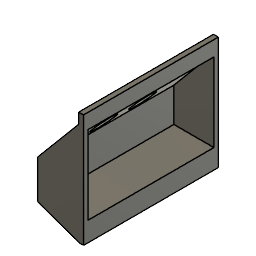
Plataforma para Sensor (Autodesk Fusion 360 design; units mm, degrees)
part number: 2026-06-29-13-53-25-750
Autodesk Fusion 360 part; units mm, degrees
sketch "Boceto1" plane through (0, 0, 0) normal (0, 1, 0) x (1, 0, 0)
  line L0 (0, 0) -> (45.0979, 0)
  line L1 (45.0979, 0) -> (45.0979, -89.5)
  line L2 (45.0979, -89.5) -> (0, -89.5)
  line L3 (0, -89.5) -> (0, 0)
  dimension "d1" = 89.5
  constraint horizontal L0
  constraint vertical L1
  constraint horizontal L2
  constraint vertical L3
  constraint coincident L0.start L3.end
  measures "d1" distance of L0.start L2.end
extrude "Extruir1" add sketch "Boceto1" along normal blind 3
sketch "Boceto2" plane through (0, 0, 0) normal (0, -1, 0) x (1, 0, 0)
  line L0 (45.0979, 89.5) -> (0, 89.5)
  line L1 (0, 89.5) -> (0, 0)
  line L2 (0, 0) -> (45.0979, 0)
  line L3 (45.0979, 0) -> (45.0979, 89.5)
  line L4 (0, 0) -> (12.1, 0)
  line L5 (12.1, 89.5) -> (0, 89.5)
  line L6 (0, 89.5) -> (0, 0)
  point P0 (12.1, 0)
  point P1 (12.1, 89.5)
  constraint horizontal L4
  constraint horizontal L5
  constraint vertical L6
  constraint coincident L1.end L2.start
  constraint coincident P0 L4.end
  constraint coincident P1 L5.start
ref_plane "PlanoDeObra1" through (12.1, 0, 44.75) normal (-0.707107, 0.707107, 0) x (0, 0, -1)
sketch "Boceto3" plane through (45.0979, 0, 0) normal (1, 0, 0) x (0, 0, -1)
  line L0 (-89.5, 0) -> (0, 0)
  line L1 (0, 0) -> (0, 3)
  line L2 (0, 3) -> (-89.5, 3)
  line L3 (-89.5, 3) -> (-89.5, 0)
  line L4 (0, 0) -> (-89.5, 0)
  line L5 (-89.5, 0) -> (-89.5, 35.5)
  line L6 (-89.5, 35.5) -> (0, 35.5)
  line L7 (0, 35.5) -> (0, 0)
  line L8 (-86.5, 3) -> (-86.5, 32.5)
  line L9 (-86.5, 32.5) -> (-3, 32.5)
  line L10 (-3, 32.5) -> (-3, 3)
  line L11 (-3, 3) -> (-86.5, 3)
  dimension "d6" = 89.5
  dimension "d7" = 35.5
  dimension "d8" = 3
  constraint horizontal L4
  constraint vertical L5
  constraint horizontal L6
  constraint vertical L7
  constraint coincident L0.end L1.start
  measures "d6" distance of L0.end L0.start
  measures "d7" distance of L0.end L6.end
extrude "Extruir2" add sketch "Boceto3" against normal blind 3 contours L2 L5 L6 L7 L8 L9 L10
sketch "Boceto4" plane through (6.05, -6.05, 0) normal (-0.707107, 0.707107, 0) x (0, 0, -1)
ref_plane "PlanoDeObra2" through (12.1, 0, 44.75) normal (-0.766044, 0.642788, 0) x (0, 0, -1)
sketch "Boceto5" plane through (7.1006, -5.9581, 0) normal (-0.766044, 0.642788, 0) x (0, 0, -1)
  line L0 (-89.5, -7.7775) -> (0, -7.7775)
  line L1 (0, -7.7775) -> (0, -54.0244)
  line L2 (0, -54.0244) -> (-89.5, -54.0244)
  line L3 (-89.5, -54.0244) -> (-89.5, -7.7775)
  dimension "d12" = 89.5
  constraint horizontal L0
  constraint vertical L1
  constraint horizontal L2
  constraint vertical L3
  measures "d12" distance of L0.start L0.end
extrude "Extruir3" add sketch "Boceto5" against normal blind 3
extrude "Extruir4" cut sketch "Boceto2" along normal blind 3
sketch "Boceto6" plane through (7.1006, -5.9581, 0) normal (-0.766044, 0.642788, 0) x (0, 0, 1)
  line L0 (0, 11.694) -> (89.5, 11.694)
  line L1 (89.5, 11.694) -> (89.5, 54.0244)
  line L2 (89.5, 54.0244) -> (0, 54.0244)
  line L3 (0, 54.0244) -> (0, 11.694)
  circle A0 centre (57.7, 26.8462) radius 7.95
  circle A1 centre (31.8, 26.8462) radius 7.95
  dimension "d18" = 15.9
  dimension "d19" = 25.9
  dimension "d20" = 15.9
  measures "d18" diameter of A0
  measures "d19" distance of A0.centre A1.centre
  measures "d20" diameter of A1
extrude "Extruir5" cut sketch "Boceto6" against normal blind 3 contours A0 | A1
sketch "Boceto7" plane through (0, 3, 0) normal (0, 1, 0) x (-1, 0, 0)
  line L0 (-14.6173, 89.5) -> (-14.6173, 0)
  line L1 (-14.6173, 0) -> (0, 0)
  line L2 (0, 0) -> (0, 89.5)
  line L3 (0, 89.5) -> (-14.6173, 89.5)
  circle A0 centre (-8, 5) radius 3.25
  circle A1 centre (-7.3086, 84.9016) radius 3.25
  dimension "d23" = 6.5
  dimension "d24" = 6.5
  measures "d23" diameter of A0
  measures "d24" diameter of A1
extrude "Extruir6" cut sketch "Boceto7" against normal blind 3 contours A0 | A1
sketch "Boceto8" plane through (0, 0, 89.5) normal (0, 0, 1) x (1, 0, 0)
  line L0 (18.5335, 3) -> (42.0979, 31.083)
  line L1 (42.0979, 31.083) -> (42.0979, 3)
  line L2 (42.0979, 3) -> (18.5335, 3)
  line L3 (12.1, 0) -> (16.0162, 0)
  line L4 (16.0162, 0) -> (45.0979, 0)
  line L5 (45.0979, 0) -> (45.0979, 35.5)
  line L6 (45.0979, 35.5) -> (42.0979, 35.5)
  line L7 (42.0979, 35.5) -> (42.0979, 35.1995)
  line L8 (42.0979, 35.1995) -> (41.8268, 35.427)
  line L9 (41.8268, 35.427) -> (14.6173, 3)
  line L10 (14.6173, 3) -> (0, 3)
  line L11 (0, 3) -> (0, 0)
  line L12 (0, 0) -> (12.1, 0)
  line L13 (18.5335, 3) -> (42.0979, 3)
  line L14 (42.0979, 31.083) -> (18.5335, 3)
  constraint coincident L0.start L2.end
  constraint coincident L1.end L2.start
  constraint coincident L0.end L1.start
extrude "Extruir7" add sketch "Boceto8" against normal blind 3 contours L0 L1 L2 L13 L14
sketch "Boceto9" plane through (0, 0, 0) normal (0, 0, -1) x (-1, 0, 0)
  line L0 (-16.0162, 0) -> (-12.1, 0)
  line L1 (-12.1, 0) -> (0, 0)
  line L2 (0, 0) -> (0, 3)
  line L3 (0, 3) -> (-14.6173, 3)
  line L4 (-14.6173, 3) -> (-41.8268, 35.427)
  line L5 (-41.8268, 35.427) -> (-42.0979, 35.1995)
  line L6 (-42.0979, 35.1995) -> (-42.0979, 35.5)
  line L7 (-42.0979, 35.5) -> (-45.0979, 35.5)
  line L8 (-45.0979, 35.5) -> (-45.0979, 0)
  line L9 (-45.0979, 0) -> (-16.0162, 0)
  line L10 (-18.5335, 3) -> (-42.0979, 3)
  line L11 (-42.0979, 3) -> (-42.0979, 31.083)
  line L12 (-42.0979, 31.083) -> (-18.5335, 3)
  line L13 (-42.0979, 3) -> (-18.5335, 3)
  line L14 (-42.0979, 31.083) -> (-42.0979, 3)
  constraint coincident L10.end L11.start
  constraint coincident L10.start L12.end
  constraint coincident L11.end L12.start
extrude "Extruir8" add sketch "Boceto9" against normal blind 3 contours L10 L11 L12 L13 L14
sketch "Boceto10" plane through (45.0979, 0, 0) normal (1, 0, 0) x (0, 0, -1)
  line L0 (-3, 3) -> (-86.5, 3)
  line L1 (-86.5, 3) -> (-86.5, 32.5)
  line L2 (-86.5, 32.5) -> (-3, 32.5)
  line L3 (-3, 32.5) -> (-3, 3)
  line L4 (0, 0) -> (0, 35.5)
  line L5 (0, 35.5) -> (-89.5, 35.5)
  line L6 (-89.5, 35.5) -> (-89.5, 0)
  line L7 (-89.5, 0) -> (0, 0)
  line L8 (0, 34) -> (-89.5, 34)
  line L9 (-89.5, 34) -> (-89.5, 49.617)
  line L10 (-89.5, 49.617) -> (0, 49.617)
  line L11 (0, 49.617) -> (0, 34)
  dimension "d31" = 89.5
  dimension "d32" = 15.617
  constraint horizontal L8
  constraint vertical L9
  constraint horizontal L10
  constraint vertical L11
  constraint coincident L4 L8.start
  measures "d31" distance of L8.start L8.end
  measures "d32" distance of L8.start L10.end
extrude "Extruir9" add sketch "Boceto10" against normal blind 3.271 contours L4 L5 L6 L8 L9 L11 | L5 L9 L10 L11
sketch "Boceto11" plane through (41.8269, 0, 0) normal (-1, 0, 0) x (0, 0, 1)
  line L0 (0, 35.4269) -> (89.5, 35.4269)
  line L1 (89.5, 35.4269) -> (89.5, 49.617)
  line L2 (89.5, 49.617) -> (0, 49.617)
  line L3 (0, 49.617) -> (0, 35.4269)
  circle A0 centre (82, 43) radius 3.25
  circle A1 centre (10, 43) radius 3.25
  dimension "d35" = 6.5
  dimension "d36" = 6.5
  measures "d35" diameter of A0
  measures "d36" diameter of A1
extrude "Extruir10" cut sketch "Boceto11" against normal blind 3.271 contours A0 | A1
extrude "Extruir11" cut 1 faces at (41.8269, 42.6813, 2.25) along direction (1, 0, 0) blind 3
extrude "Extruir12" cut 1 faces at (44.8269, 42.6813, 2.25) along direction (1, 0, 0) blind 1
sketch "Boceto12" plane through (45.0979, 0, 0) normal (1, 0, 0) x (0, 0, -1)
  line L0 (-3, 3) -> (-86.5, 3)
  line L1 (-86.5, 3) -> (-86.5, 32.5)
  line L2 (-86.5, 32.5) -> (-3, 32.5)
  line L3 (-3, 32.5) -> (-3, 3)
  line L4 (0, 35.4269) -> (-89.5, 35.4269)
  line L5 (-89.5, 35.4269) -> (-89.5, 0)
  line L6 (-89.5, 0) -> (0, 0)
  line L7 (0, 0) -> (0, 35.4269)
  line L8 (0, 35.4269) -> (0, 42.4269)
  line L9 (0, 42.4269) -> (-10, 42.4269)
  line L10 (-10, 42.4269) -> (-10, -32.5731)
  line L11 (-10, -32.5731) -> (0, -32.5731)
  line L12 (0, -32.5731) -> (0, 42.4269)
  dimension "d43" = 7
  dimension "d44" = 10
  dimension "d45" = 75
  constraint coincident L4.start L7.end
  constraint perpendicular L4 L8
  constraint horizontal L9
  constraint vertical L10
  constraint horizontal L11
  constraint vertical L12
  measures "d43" distance of L4.start L8.end
  measures "d44" distance of L8.end L9.end
  measures "d45" distance of L8.end L11.end
extrude "Extruir13" add sketch "Boceto12" against normal blind 3.271 contours L0 L2 L3 L4 L6 L7 L10 L12 | L0 L2 L3 L10 | L6 L10 L11 L12 | L4 L8 L9 L10 L12
sketch "Boceto13" plane through (45.0979, 0, 0) normal (1, 0, 0) x (0, 0, -1)
  line L0 (-10, 3) -> (-86.5, 3)
  line L1 (-86.5, 3) -> (-86.5, 32.5)
  line L2 (-86.5, 32.5) -> (-10, 32.5)
  line L3 (-10, 32.5) -> (-10, 3)
  line L4 (0, -32.5731) -> (0, 42.4269)
  line L5 (0, 42.4269) -> (-10, 42.4269)
  line L6 (-10, 42.4269) -> (-10, 35.4269)
  line L7 (-10, 35.4269) -> (-89.5, 35.4269)
  line L8 (-89.5, 35.4269) -> (-89.5, 0)
  line L9 (-89.5, 0) -> (-10, 0)
  line L10 (-10, 0) -> (-10, -32.5731)
  line L11 (-10, -32.5731) -> (0, -32.5731)
  line L12 (-89.5, 35.4269) -> (-89.5, 42.4269)
  line L13 (-89.5, 42.4269) -> (-79.5, 42.4269)
  line L14 (-79.5, 42.4269) -> (-79.5, -32.5731)
  line L15 (-79.5, -32.5731) -> (-89.5, -32.5731)
  line L16 (-89.5, -32.5731) -> (-89.5, 42.4269)
  dimension "d48" = 7
  dimension "d49" = 10
  dimension "d50" = 75
  constraint coincident L7.end L8.start
  constraint perpendicular L7 L12
  constraint horizontal L13
  constraint vertical L14
  constraint horizontal L15
  constraint vertical L16
  measures "d48" distance of L7.end L12.end
  measures "d49" distance of L12.end L13.end
  measures "d50" distance of L12.end L15.end
extrude "Extruir14" add sketch "Boceto13" against normal blind 3.271 contours L0 L1 L2 L7 L8 L9 L14 L16 | L0 L1 L2 L14 | L9 L14 L15 L16 | L7 L12 L13 L14 L16
sketch "Boceto14" plane through (45.0979, 0, 0) normal (1, 0, 0) x (0, 0, -1)
  line L0 (-79.5, 0) -> (-10, 0)
  line L1 (-10, 0) -> (-10, -32.5731)
  line L2 (-10, -32.5731) -> (0, -32.5731)
  line L3 (0, -32.5731) -> (0, 42.4269)
  line L4 (0, 42.4269) -> (-10, 42.4269)
  line L5 (-10, 42.4269) -> (-10, 35.4269)
  line L6 (-10, 35.4269) -> (-79.5, 35.4269)
  line L7 (-79.5, 35.4269) -> (-79.5, 42.4269)
  line L8 (-79.5, 42.4269) -> (-89.5, 42.4269)
  line L9 (-89.5, 42.4269) -> (-89.5, -32.5731)
  line L10 (-89.5, -32.5731) -> (-79.5, -32.5731)
  line L11 (-79.5, -32.5731) -> (-79.5, 0)
  line L12 (-79.5, 3) -> (-79.5, 32.5)
  line L13 (-79.5, 32.5) -> (-10, 32.5)
  line L14 (-10, 32.5) -> (-10, 3)
  line L15 (-10, 3) -> (-79.5, 3)
  line L16 (0, -32.5731) -> (-89.5, -32.5731)
  line L17 (-89.5, -32.5731) -> (-89.5, -22.5731)
  line L18 (-89.5, -22.5731) -> (0, -22.5731)
  line L19 (0, -22.5731) -> (0, -32.5731)
  line L20 (-89.5, 42.4269) -> (0, 42.4269)
  line L21 (0, 42.4269) -> (0, 35.4269)
  line L22 (0, 35.4269) -> (-89.5, 35.4269)
  line L23 (-89.5, 35.4269) -> (-89.5, 42.4269)
  dimension "d53" = 10
  constraint horizontal L16
  constraint vertical L17
  constraint horizontal L18
  constraint vertical L19
  constraint coincident L2.end L3.start
  constraint horizontal L20
  constraint vertical L21
  constraint horizontal L22
  constraint vertical L23
  constraint coincident L3 L21.end
  constraint coincident L8.end L9.start
  measures "d53" distance of L2.end L18.end
extrude "Extruir15" add sketch "Boceto14" against normal blind 3.271 contours L1 L11 L16 L18 | L5 L6 L7 L20 L22
sketch "Boceto15" plane through (0, 3, 0) normal (0, 1, 0) x (-1, 0, 0)
  circle A0 centre (-7.3086, 84.9016) radius 3.25
  circle A1 centre (-8, 5) radius 3.25
  line L0 (-14.6173, 89.5) -> (-14.6173, 0)
  line L1 (-14.6173, 0) -> (0, 0)
  line L2 (0, 0) -> (0, 89.5)
  line L3 (0, 89.5) -> (-14.6173, 89.5)
  line L4 (0, 0) -> (-14.6173, 0)
  line L5 (-14.6173, 0) -> (-14.6173, 89.5)
  line L6 (-14.6173, 89.5) -> (0, 89.5)
  line L7 (0, 89.5) -> (0, 0)
  constraint horizontal L4
  constraint vertical L5
  constraint horizontal L6
  constraint vertical L7
  constraint coincident L0.start L3.end
  constraint coincident L1.end L2.start
extrude "Extruir16" cut sketch "Boceto15" against normal blind 3.271
extrude "Extruir17" add 1 faces at (41.8269, -29.2397, 33.1667) along direction (-1, 0, 0) blind 27
sketch "Boceto16" plane through (14.8269, 0, 0) normal (-1, 0, 0) x (0, 0, 1)
  line L0 (10, 0) -> (0, 0)
  line L1 (0, 0) -> (0, -32.5731)
  line L2 (0, -32.5731) -> (89.5, -32.5731)
  line L3 (89.5, -32.5731) -> (89.5, 0)
  line L4 (89.5, 0) -> (79.5, 0)
  line L5 (79.5, 0) -> (79.5, -22.5731)
  line L6 (79.5, -22.5731) -> (10, -22.5731)
  line L7 (10, -22.5731) -> (10, 0)
  line L8 (10, -22.5731) -> (79.5, -22.5731)
  line L9 (79.5, -22.5731) -> (79.5, 0)
  line L10 (79.5, 0) -> (10, 0)
  line L11 (10, 0) -> (10, -22.5731)
  constraint horizontal L8
  constraint vertical L9
  constraint horizontal L10
  constraint vertical L11
  constraint coincident L4.end L5.start
  constraint coincident L6.end L7.start
extrude "Extruir18" add sketch "Boceto16" against normal blind 3 contours L5 L6 L7 L8 L9 L10 L11
extrude "Extruir19" cut 1 faces at (36.0076, -22.5731, 56.3333) along direction (0, -1, 0) blind 7
extrude "Extruir20" cut 1 faces at (26.9173, 0, 56.3333) along direction (0, 1, 0) blind 3
extrude "Extruir21" cut 1 faces at (34.9173, -18.7154, 10) along direction (0, 0, -1) blind 7
extrude "Extruir22" cut 1 faces at (34.9173, -18.7154, 79.5) along direction (0, 0, 1) blind 7
sketch "Boceto17" plane through (45.0979, 0, 0) normal (1, 0, 0) x (0, 0, -1)
  line L0 (-89.5, -32.5731) -> (0, -32.5731)
  line L1 (0, -32.5731) -> (0, 42.4269)
  line L2 (0, 42.4269) -> (-89.5, 42.4269)
  line L3 (-89.5, 42.4269) -> (-89.5, -32.5731)
  line L4 (-3, -29.5731) -> (-86.5, -29.5731)
  line L5 (-86.5, -29.5731) -> (-86.5, 32.5)
  line L6 (-86.5, 32.5) -> (-3, 32.5)
  line L7 (-3, 32.5) -> (-3, -29.5731)
  line L8 (0, 42.4269) -> (-10, 42.4269)
  line L9 (-10, 42.4269) -> (-10, -32.5731)
  line L10 (-10, -32.5731) -> (0, -32.5731)
  line L11 (0, -32.5731) -> (0, 42.4269)
  line L12 (-89.5, 42.4269) -> (-79.5, 42.4269)
  line L13 (-79.5, 42.4269) -> (-79.5, -32.5731)
  line L14 (-79.5, -32.5731) -> (-89.5, -32.5731)
  line L15 (-89.5, -32.5731) -> (-89.5, 42.4269)
  dimension "d70" = 10
  dimension "d71" = 75
  dimension "d72" = 10
  dimension "d73" = 75
  constraint horizontal L8
  constraint vertical L9
  constraint horizontal L10
  constraint vertical L11
  constraint coincident L1.end L2.start
  constraint horizontal L12
  constraint vertical L13
  constraint horizontal L14
  constraint vertical L15
  constraint coincident L2.end L3.start
  measures "d70" distance of L1.end L8.end
  measures "d71" distance of L1.end L0.end
  measures "d72" distance of L2.end L12.end
  measures "d73" distance of L2.end L0.start
extrude "Extruir23" add sketch "Boceto17" against normal blind 3 contours L0 L2 L3 L4 L5 L6 L12 L13 L14 L15 | L0 L1 L2 L4 L6 L7 L8 L9 L10 L11 | L4 L5 L6 L13 | L4 L6 L7 L9
extrude "Extruir24" add 1 faces at (17.8269, -7.8577, 30.8333) along direction (1, 0, 0) blind 0.707
extrude "Extruir25" add 1 faces at (14.8269, -10.8577, 59.6667) along direction (-1, 0, 0) blind 0.21
sketch "Boceto18" plane through (45.0979, 0, 0) normal (1, 0, 0) x (0, 0, -1)
  line L0 (-79.5, 32.5) -> (-10, 32.5)
  line L1 (-10, 32.5) -> (-10, -29.5731)
  line L2 (-10, -29.5731) -> (-79.5, -29.5731)
  line L3 (-79.5, -29.5731) -> (-79.5, 32.5)
  line L4 (0, 42.4269) -> (-89.5, 42.4269)
  line L5 (-89.5, 42.4269) -> (-89.5, -32.5731)
  line L6 (-89.5, -32.5731) -> (0, -32.5731)
  line L7 (0, -32.5731) -> (0, 42.4269)
  line L8 (-89.5, -32.5731) -> (0, -32.5731)
  line L9 (0, -32.5731) -> (0, -22.5731)
  line L10 (0, -22.5731) -> (-89.5, -22.5731)
  line L11 (-89.5, -22.5731) -> (-89.5, -32.5731)
  dimension "d80" = 89.5
  dimension "d81" = 10
  constraint horizontal L8
  constraint vertical L9
  constraint horizontal L10
  constraint vertical L11
  constraint coincident L5.end L6.start
  measures "d80" distance of L5.end L6.end
  measures "d81" distance of L5.end L10.end
extrude "Extruir26" add sketch "Boceto18" against normal blind 3 contours L1 L2 L3 L10
sketch "Boceto19" plane through (14.6169, 0, 0) normal (-1, 0, 0) x (0, 0, 1)
  line L0 (89.5, 0) -> (0, 0)
  line L1 (0, 0) -> (0, -32.5731)
  line L2 (0, -32.5731) -> (89.5, -32.5731)
  line L3 (89.5, -32.5731) -> (89.5, 0)
  line L4 (0, -32.5731) -> (89.5, -32.5731)
  line L5 (89.5, -32.5731) -> (89.5, -22.5731)
  line L6 (89.5, -22.5731) -> (0, -22.5731)
  line L7 (0, -22.5731) -> (0, -32.5731)
  dimension "d84" = 89.5
  dimension "d85" = 10
  constraint horizontal L4
  constraint vertical L5
  constraint horizontal L6
  constraint vertical L7
  constraint coincident L1.end L2.start
  measures "d84" distance of L1.end L2.end
  measures "d85" distance of L1.end L6.end
extrude "Extruir27" cut sketch "Boceto19" against normal blind 27.841 contours L1 L2 L3 L4 L5 L6 L7
sketch "Boceto20" plane through (0, -22.5731, 0) normal (0, -1, 0) x (1, 0, 0)
  line L0 (42.0979, 79.5) -> (42.4579, 79.5)
  line L1 (42.4579, 79.5) -> (42.4579, 89.5)
  line L2 (42.4579, 89.5) -> (14.6169, 89.5)
  line L3 (14.6169, 89.5) -> (14.6169, 0)
  line L4 (14.6169, 0) -> (42.4579, 0)
  line L5 (42.4579, 0) -> (42.4579, 10)
  line L6 (42.4579, 10) -> (42.0979, 10)
  line L7 (42.0979, 10) -> (42.0979, 3)
  line L8 (42.0979, 3) -> (18.5339, 3)
  line L9 (18.5339, 3) -> (18.5339, 86.5)
  line L10 (18.5339, 86.5) -> (42.0979, 86.5)
  line L11 (42.0979, 86.5) -> (42.0979, 79.5)
  line L12 (42.4579, 0) -> (18.5339, 0)
  line L13 (18.5339, 0) -> (18.5339, 86.5)
  line L14 (18.5339, 86.5) -> (42.4579, 86.5)
  line L15 (42.4579, 86.5) -> (42.4579, 0)
  line L16 (42.4579, 0) -> (18.5339, 0)
  line L17 (18.5339, 0) -> (18.5339, 86.5)
  line L18 (18.5339, 86.5) -> (42.4579, 86.5)
  line L19 (42.4579, 86.5) -> (42.4579, 0)
  constraint horizontal L12
  constraint vertical L13
  constraint horizontal L14
  constraint vertical L15
  constraint coincident L9.end L10.start
  constraint coincident L4.end L5.start
  constraint horizontal L16
  constraint vertical L17
  constraint horizontal L18
  constraint vertical L19
extrude "Extruir28" add sketch "Boceto20" against normal blind 3 contours L0 L6 L7 L8 L9 L10 L11 L13 L14 L15 L17 L18 L19
extrude "Extruir29" add 1 faces at (42.4579, -21.5731, 56.3333) along direction (1, 0, 0) blind 2.64
extrude "Extruir30" cut 1 faces at (44.0979, 14.67, 10) along direction (0, 0, -1) blind 7
extrude "Extruir31" cut 1 faces at (44.0979, 14.67, 79.5) along direction (0, 0, 1) blind 7
sketch "Boceto21" plane through (0, 0, 0) normal (0, 0, -1) x (-1, 0, 0)
  line L0 (-42.4579, -32.5731) -> (-42.4579, -22.5731)
  line L1 (-42.4579, -22.5731) -> (-14.6169, -22.5731)
  line L2 (-14.6169, -22.5731) -> (-14.6169, 0)
  line L3 (-14.6169, 0) -> (-14.6173, 0)
  line L4 (-14.6173, 0) -> (-14.6173, 3)
  line L5 (-14.6173, 3) -> (-41.8268, 35.427)
  line L6 (-41.8268, 35.427) -> (-41.8269, 35.4269)
  line L7 (-41.8269, 35.4269) -> (-41.8269, 42.4269)
  line L8 (-41.8269, 42.4269) -> (-45.0979, 42.4269)
  line L9 (-45.0979, 42.4269) -> (-45.0979, -32.5731)
  line L10 (-45.0979, -32.5731) -> (-42.4579, -32.5731)
  line L11 (-42.4579, -32.5731) -> (-14.6169, -22.5731)
  line L12 (-42.4579, -22.5731) -> (-42.4579, -32.5731)
  constraint coincident L0.start L10.end
  constraint coincident L1.end L2.start
  constraint coincident L0.end L1.start
extrude "Extruir32" add sketch "Boceto21" against normal blind 89.5 contours L0 L1 L11 L12
equation "d18 = 7.95 mm + 7.95 mm"
equation "d19 = 7.95 mm + 10 mm + 7.95 mm"
equation "d32 = 14.617 mm + 1 mm"
